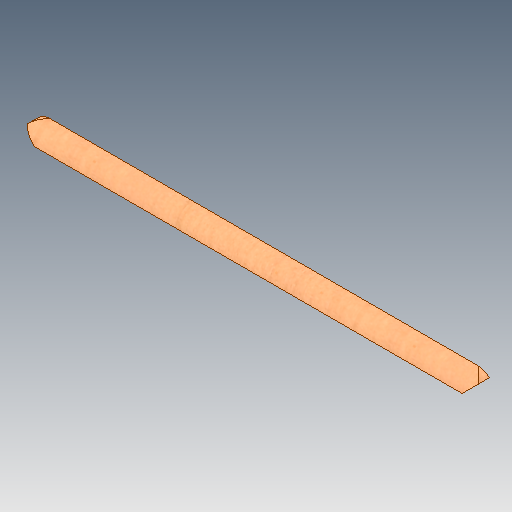
# Autodesk Inventor part: frontBackMoulding
Saved by Autodesk Inventor 2018.2 (Build 222227000, 227)
## iProperties
Created: 2016-04-01
Part Number: frontBackMoulding
Material: Wood (Cherry)
Document SubType Name: Modeling
Designer: sawai
Density: 0.63 g/cm^3
Appearance: Cherry - Natural Low Gloss
Author: sawai
Autodesk Inventor part; units mm, degrees
ref_plane "YZ Plane" through (0, 0, 0) normal (1, 0, 0) x (0, 1, 0)
ref_plane "XZ Plane" through (0, 0, 0) normal (0, 1, 0) x (-1, 0, 0)
ref_plane "XY Plane" through (0, 0, 0) normal (0, 0, 1) x (1, 0, 0)
sketch "Sketch1" plane through (0, 0, 0) normal (1, 0, 0) x (0, 1, 0)
  line L0 (-6.35, 6.35) -> (6.35, 6.35)
  line L1 (6.35, 6.35) -> (6.35, -6.35)
  line L2 (6.35, -6.35) -> (-6.35, -6.35)
  line L3 (-6.35, -6.35) -> (-6.35, 6.35)
  line L4 (-6.35, 6.35) -> (6.35, -6.35) construction
  line L5 (6.35, 6.35) -> (-6.35, -6.35) construction
  point P0 (0, 0)
  dimension "d0" = 12.7
  dimension "d1" = 12.7
  constraints: 12 end point, 2 midpoint, 2 parallel, 1 horizontal, 1 perpendicular
  measures "d0" distance of L1.end L2.end
  measures "d1" distance of L0.end L1.end
extrude "Extrusion1" add sketch "Sketch1" along normal mid plane 365.4
fillet "Fillet1" radius 12.7 3 edges at (0, 6.35, 6.35) (-182.7, 6.35, 0) (182.7, 6.35, 0)
chamfer "Chamfer1" distance 6.35 angle 45 1 edges at (0, -6.35, -6.35)
sketch "Sketch2" plane through (0, 0, 0) normal (0, 0, 1) x (1, 0, 0)
  line L0 (-182.7, -6.35) -> (182.7, -6.35) projected
  line L1 (170, 6.35) -> (-170, 6.35) projected
  line L2 (-182.7, -6.35) -> (-182.7, 6.35)
  line L3 (-182.7, 6.35) -> (-170, -6.35)
  line L4 (-182.7, 6.35) -> (-170, 6.35) construction
  point P0 (0, 0)
  dimension "d11" = 45
  constraints: 6 end point, 1 horizontal, 1 point on line, 1 vertical
  measures "d11" angle of L0 L3
extrude "Extrusion2" cut sketch "Sketch2" along normal through all both and the other way through all
mirror "Mirror1" about plane through (0, 0, 0) normal (1, 0, 0) of "Extrusion2"
sketch "Sketch3" plane through (0, 0, 0) normal (1, 0, 0) x (0, 1, 0)
  line L0 (-6.35, 6.35) -> (-6.35, 6.35) projected
  line L1 (-6.35, 0) -> (-6.35, 6.35) projected
  line L2 (0, -6.35) -> (-6.35, 0) projected
  line L3 (2.6303, -6.35) -> (0, -6.35) projected
  line L4 (2.6303, 2.6303) -> (2.6303, -6.35) projected
  arc A0 (2.6303, 2.6303) -> (-6.35, 6.35) centre (-6.35, -6.35) ccw projected
  circle A1 centre (0, -6.35) radius 1.5875
  line L5 (6.35, -6.35) -> (2.6303, -6.35) projected
  point P0 (0, 0)
  dimension "d14" = 3.175
  dimension "d15" = 6.35
  constraints: 1 centre point, 1 point on line
  measures "d14" diameter of A1
  measures "d15" distance of L5.start A1.centre
extrude "Extrusion3" cut sketch "Sketch3" along normal through all both and the other way through all contours A1 L3 L2 | L2 L3 A1
equation "\"d0\" = facingThickness"
equation "\"d1\" = facingThickness"
equation "\"d7\" = 0.999999 * facingThickness"
equation "\"d4\" = 0.5 * facingThickness"
equation "\"d14\" = 0.25 * facingThickness"
equation "\"d15\" = 0.5 * facingThickness"
equation "\"facingThickness\" = 12.7"
equation "\"facingGasketThickness\" = 1.5875"
body "Solid1"
